Bench Vice_ (Autodesk Fusion 360 archive; units mm, degrees)
design "Screw Bar"
Autodesk Fusion 360 part; units mm, degrees
sketch "Sketch1" plane through (0, 0, 0) normal (0, 0, 1) x (1, 0, 0)
  line L0 (0, 0) -> (84, 0)
  line L1 (84, 0) -> (84, 3)
  line L2 (84, 3) -> (94, 3)
  line L3 (94, 3) -> (94, 5)
  line L4 (94, 5) -> (-10, 5)
  line L5 (-10, 5) -> (-10, 3)
  line L6 (-10, 3) -> (0, 3)
  line L7 (0, 3) -> (0, 0)
  constraint coincident L0.start L7.end
  constraint horizontal L0
  constraint perpendicular L0 L1
  constraint perpendicular L1 L2
  constraint vertical L3
  constraint perpendicular L3 L4
  constraint perpendicular L4 L5
  constraint perpendicular L5 L6
revolve "Revolve1" add sketch "Sketch1" angle 360 about axis through (94, 5, 0) along (-1, 0, 0)

design "Untitled"
Autodesk Fusion 360 part; units mm, degrees
sketch "Sketch1" plane through (0, 0, 0) normal (0, 1, 0) x (1, 0, 0)
  line L0 (0, 0) -> (144, 0)
  line L1 (144, 0) -> (144, -16)
  line L2 (144, -16) -> (0, -16)
  line L3 (0, -16) -> (0, 0)
  line L4 (0, -16) -> (26, -16)
  line L5 (26, -16) -> (26, -52)
  line L6 (26, -52) -> (16, -52)
  line L7 (0, -36) -> (0, -16)
  line L8 (144, -16) -> (122, -16)
  line L9 (122, -16) -> (122, -52)
  line L10 (122, -52) -> (144, -52)
  line L11 (144, -52) -> (144, -16)
  line L12 (0, -36) -> (16, -52)
  dimension "d1" = 144
  dimension "d2" = 16
  dimension "d3" = 26
  dimension "d5" = 22
  dimension "d6" = 36
  constraint horizontal L0
  constraint vertical L1
  constraint horizontal L2
  constraint vertical L3
  constraint coincident L0.start L3.end
  constraint horizontal L4
  constraint vertical L5
  constraint horizontal L6
  constraint vertical L7
  constraint horizontal L8
  constraint vertical L9
  constraint horizontal L10
  constraint vertical L11
  measures "d1" distance of L0.start L0.end
  measures "d2" distance of L0.start L2.end
  measures "d3" distance of L2.end L4.end
  measures "d5" distance of L1.end L8.end
  measures "d6" distance of L1.end L10.end
extrude "Extrude1" add sketch "Sketch1" along normal blind 64 makes body 1
sketch "Sketch2" plane through (144, 0, 0) normal (1, 0, 0) x (0, 1, 0)
  line L0 (0, 52) -> (0, 0)
  line L1 (0, 0) -> (64, 0)
  line L2 (64, 0) -> (64, 52)
  line L3 (64, 52) -> (0, 52)
  line L4 (16, 9) -> (16, 0)
  line L5 (48, 9) -> (48, 0)
  line L6 (16, 0) -> (16, 9)
  line L7 (24, 16) -> (40, 16)
  line L8 (24, 16) -> (24, 9)
  line L9 (40, 16) -> (40, 9)
  line L10 (16, 9) -> (24, 9)
  line L11 (40, 9) -> (48, 9)
  constraint coincident L1 L4.end
  constraint perpendicular L1 L4
  constraint coincident L1 L5.end
  constraint perpendicular L1 L5
  constraint perpendicular L5 L7
  constraint perpendicular L1 L8
  constraint perpendicular L1 L9
  constraint perpendicular L2 L10
  constraint collinear L10 L11
extrude "Extrude2" cut sketch "Sketch2" against normal blind 170 contours L1 L4 L5 L6 L7 L8 L9 L10 L11 bodies 1
sketch "Sketch3" plane through (144, 0, 0) normal (1, 0, 0) x (0, 1, 0)
  line L0 (48, 9) -> (48, 0)
  line L1 (48, 0) -> (64, 0)
  line L2 (64, 0) -> (64, 52)
  line L3 (64, 52) -> (0, 52)
  line L4 (0, 52) -> (0, 0)
  line L5 (0, 0) -> (16, 0)
  line L6 (16, 0) -> (16, 9)
  line L7 (16, 9) -> (24, 9)
  line L8 (24, 9) -> (24, 16)
  line L9 (24, 16) -> (40, 16)
  line L10 (40, 16) -> (40, 9)
  line L11 (40, 9) -> (48, 9)
  circle A0 centre (32, 36) radius 8
  line L12 (46.5857, 42.577) -> (58.5699, 16)
  line L13 (17.4559, 42.6685) -> (4.6049, 16)
  arc A1 (46.5857, 42.577) -> (17.4559, 42.6685) centre (32, 36) ccw
  line L14 (24, 16) -> (40, 16)
  line L15 (4.6049, 16) -> (0, 16)
  line L16 (58.5699, 16) -> (64, 16)
  dimension "d22" = 50
  dimension "d23" = 25.728
  dimension "d25" = 24.272
  constraint coincident L8.end L9.start
  constraint perpendicular L2 L14
  constraint concentric A0 A1
  constraint tangent L12 A1
  constraint coincident L12.end L14
  constraint perpendicular L4 L15
  constraint coincident L2 L16.end
  constraint perpendicular L2 L16
  measures "d22" angle of L12 L13
  measures "d23" angle of L4 L13
  measures "d25" angle of L2 L12
extrude "Extrude3" cut sketch "Sketch3" against normal blind 35 contours L2 L3 L12 A1 L16 | L3 L4 L13 A1 L15 | A0 bodies 1
fillet "Fillet1" radius 3 1 edges at (133, 4.6049, 16) on bodies 1
fillet "Fillet2" radius 3 1 edges at (133, 58.5699, 16) on bodies 1
sketch "Sketch4" plane through (0, 0, 0) normal (0, 1, 0) x (1, 0, 0)
hole "Hole1" at (105.944, 10.2209, 0) direction (0, 0, 1) diameter 6 depth 10 tip angle 118 bodies 1
pattern_linear "R-Pattern1" count 2 spacing 70 along (-1, 0, 0) count 2 spacing 44 along (0, 1, 0) of "Hole1"
sketch "Sketch5" plane through (26, 0, 0) normal (1, 0, 0) x (0, 1, 0)
  line L0 (0, 52) -> (0, 16)
  line L1 (0, 16) -> (24, 16)
  line L2 (40, 16) -> (64, 16)
  line L3 (64, 16) -> (64, 52)
  line L4 (64, 52) -> (0, 52)
  circle A0 centre (32, 34) radius 6
  circle A1 centre (32, 34) radius 16.0001
  line L5 (20.7258, 45.3532) -> (0, 24.7716)
  line L6 (44.2406, 44.3039) -> (64, 24.682)
  line L7 (24, 16) -> (24, 9)
  line L8 (24, 9) -> (40, 9)
  line L9 (40, 9) -> (40, 16)
  dimension "d47" = 45.2
  dimension "d48" = 45.2
  constraint concentric A0 A1
  constraint tangent A1 L5
  constraint coincident A1 L6.start
  constraint coincident A1 L5.start
  constraint coincident L0 L5.end
  constraint coincident L3 L6.end
  constraint coincident L1.end L7.start
  constraint perpendicular L1 L7
  constraint perpendicular L7 L8
  constraint coincident L2.start L9.end
  measures "d47" angle of L0 L5
  measures "d48" angle of L3 L6
sketch "Sketch6" plane through (0, 0, 9) normal (0, 0, -1) x (1, 0, 0)
sketch "Sketch7" plane through (-18, 0, 18) normal (-0.707107, 0, 0.707107) x (0, -1, 0)
  line L0 (0, 25.4558) -> (0, 48.0833)
  line L1 (0, 48.0833) -> (-64, 48.0833)
  line L2 (-64, 48.0833) -> (-64, 25.4558)
  line L3 (-64, 25.4558) -> (0, 25.4558)
sketch "Sketch8" plane through (0, 0, 11) normal (0, 0, -1) x (1, 0, 0)
extrude "Extrude1'" add 1 faces at (26, 34.6667, 40) along direction (1, 0, 0) blind 10 separate body on bodies 1 makes body 2 in component "Component"
sketch "Sketch9" plane through (36, 0, 0) normal (1, 0, 0) x (0, 1, 0)
  line L0 (0, 52) -> (0, 16)
  line L1 (0, 16) -> (64, 16)
  line L2 (64, 16) -> (64, 52)
  line L3 (64, 52) -> (0, 52)
  circle A0 centre (32, 36) radius 6
  circle A1 centre (32, 36) radius 16
  line L4 (0, 16) -> (0, 26)
  line L5 (0, 26) -> (4, 26)
  line L6 (4, 26) -> (19.3557, 45.8041)
  line L7 (60, 26) -> (44.6443, 45.8041)
  line L8 (64, 26) -> (60, 26)
  line L9 (64, 16) -> (64, 26)
  line L10 (24, 16) -> (24, 9)
  line L11 (24, 9) -> (40, 9)
  line L12 (40, 9) -> (40, 16)
  dimension "d81" = 12
  dimension "d82" = 32
  constraint concentric A0 A1
  constraint coincident L0.end L1.start
  constraint perpendicular L1 L4
  constraint horizontal L5
  constraint coincident A1 L6.end
  constraint tangent A1 L6
  constraint coincident L1 L10.start
  constraint perpendicular L1 L10
  constraint perpendicular L10 L11
  constraint coincident L1 L12.end
  constraint perpendicular L1 L12
  measures "d81" diameter of A0
  measures "d82" diameter of A1
extrude "Extrude2'" add sketch "Sketch9" along normal blind 32 contours L0 L1 L2 A1 L4 L5 L6 L7 L8 L9 | A1 | L1 L10 L11 L12 bodies 2 in component "Component"
sketch "Sketch10" plane through (26, 0, 0) normal (1, 0, 0) x (0, 1, 0)
component "Component" placed x (1, 0, 0) y (0, 1, 0) z (0, 0, 1) at (6, 0, 0)
hidden bodies 1

design "Bench Vice" references "Untitled", "Bench Vice", "Jaw Screw", "Screw Bar"
Autodesk Fusion 360 part; units mm, degrees
sketch "Sketch1" plane through (0, 0, 0) normal (0, 1, 0) x (1, 0, 0)
  line L0 (0, 0) -> (144, 0)
  line L1 (144, 0) -> (144, -16)
  line L2 (144, -16) -> (0, -16)
  line L3 (0, -16) -> (0, 0)
  line L4 (0, -16) -> (26, -16)
  line L5 (26, -16) -> (26, -52)
  line L6 (26, -52) -> (16, -52)
  line L7 (0, -36) -> (0, -16)
  line L8 (144, -16) -> (122, -16)
  line L9 (122, -16) -> (122, -52)
  line L10 (122, -52) -> (144, -52)
  line L11 (144, -52) -> (144, -16)
  line L12 (0, -36) -> (16, -52)
  dimension "d1" = 144
  dimension "d2" = 16
  dimension "d3" = 26
  dimension "d5" = 22
  dimension "d6" = 36
  constraint horizontal L0
  constraint vertical L1
  constraint horizontal L2
  constraint vertical L3
  constraint coincident L0.start L3.end
  constraint horizontal L4
  constraint vertical L5
  constraint horizontal L6
  constraint vertical L7
  constraint horizontal L8
  constraint vertical L9
  constraint horizontal L10
  constraint vertical L11
  measures "d1" distance of L0.start L0.end
  measures "d2" distance of L0.start L2.end
  measures "d3" distance of L2.end L4.end
  measures "d5" distance of L1.end L8.end
  measures "d6" distance of L1.end L10.end
extrude "Extrude1" add sketch "Sketch1" along normal blind 64
sketch "Sketch2" plane through (144, 0, 0) normal (1, 0, 0) x (0, 1, 0)
  line L0 (0, 52) -> (0, 0)
  line L1 (0, 0) -> (64, 0)
  line L2 (64, 0) -> (64, 52)
  line L3 (64, 52) -> (0, 52)
  line L4 (16, 9) -> (16, 0)
  line L5 (48, 9) -> (48, 0)
  line L6 (16, 0) -> (16, 9)
  line L7 (24, 16) -> (40, 16)
  line L8 (24, 16) -> (24, 9)
  line L9 (40, 16) -> (40, 9)
  line L10 (16, 9) -> (24, 9)
  line L11 (40, 9) -> (48, 9)
  constraint coincident L1 L4.end
  constraint perpendicular L1 L4
  constraint coincident L1 L5.end
  constraint perpendicular L1 L5
  constraint perpendicular L5 L7
  constraint perpendicular L1 L8
  constraint perpendicular L1 L9
  constraint perpendicular L2 L10
  constraint collinear L10 L11
extrude "Extrude2" cut sketch "Sketch2" against normal blind 170 contours L1 L4 L5 L6 L7 L8 L9 L10 L11
sketch "Sketch3" plane through (144, 0, 0) normal (1, 0, 0) x (0, 1, 0)
  line L0 (48, 9) -> (48, 0)
  line L1 (48, 0) -> (64, 0)
  line L2 (64, 0) -> (64, 52)
  line L3 (64, 52) -> (0, 52)
  line L4 (0, 52) -> (0, 0)
  line L5 (0, 0) -> (16, 0)
  line L6 (16, 0) -> (16, 9)
  line L7 (16, 9) -> (24, 9)
  line L8 (24, 9) -> (24, 16)
  line L9 (24, 16) -> (40, 16)
  line L10 (40, 16) -> (40, 9)
  line L11 (40, 9) -> (48, 9)
  circle A0 centre (32, 36) radius 8
  line L12 (46.5857, 42.577) -> (58.5699, 16)
  line L13 (17.4559, 42.6685) -> (4.6049, 16)
  arc A1 (46.5857, 42.577) -> (17.4559, 42.6685) centre (32, 36) ccw
  line L14 (24, 16) -> (40, 16)
  line L15 (4.6049, 16) -> (0, 16)
  line L16 (58.5699, 16) -> (64, 16)
  dimension "d22" = 50
  dimension "d23" = 25.728
  dimension "d25" = 24.272
  constraint coincident L8.end L9.start
  constraint perpendicular L2 L14
  constraint concentric A0 A1
  constraint tangent L12 A1
  constraint coincident L12.end L14
  constraint perpendicular L4 L15
  constraint coincident L2 L16.end
  constraint perpendicular L2 L16
  measures "d22" angle of L12 L13
  measures "d23" angle of L4 L13
  measures "d25" angle of L2 L12
extrude "Extrude3" cut sketch "Sketch3" against normal blind 35 contours L2 L3 L12 A1 L16 | L3 L4 L13 A1 L15 | A0
fillet "Fillet1" radius 3 1 edges at (133, 4.6049, 16)
fillet "Fillet2" radius 3 1 edges at (133, 58.5699, 16)
sketch "Sketch4" plane through (0, 0, 0) normal (0, 1, 0) x (1, 0, 0)
hole "Hole1" at (105.944, 10.2209, 0) direction (0, 0, 1) diameter 6 depth 10 tip angle 118
pattern_linear "R-Pattern1" count 2 spacing 70 along (-1, 0, 0) count 2 spacing 44 along (0, 1, 0) of "Hole1"
sketch "Sketch5" plane through (26, 0, 0) normal (1, 0, 0) x (0, 1, 0)
  line L0 (0, 52) -> (0, 16)
  line L1 (0, 16) -> (24, 16)
  line L2 (40, 16) -> (64, 16)
  line L3 (64, 16) -> (64, 52)
  line L4 (64, 52) -> (0, 52)
  circle A0 centre (32, 34) radius 6
  circle A1 centre (32, 34) radius 16.0001
  line L5 (20.7258, 45.3532) -> (0, 24.7716)
  line L6 (44.2406, 44.3039) -> (64, 24.682)
  line L7 (24, 16) -> (24, 9)
  line L8 (24, 9) -> (40, 9)
  line L9 (40, 9) -> (40, 16)
  dimension "d47" = 45.2
  dimension "d48" = 45.2
  constraint concentric A0 A1
  constraint tangent A1 L5
  constraint coincident A1 L6.start
  constraint coincident A1 L5.start
  constraint coincident L0 L5.end
  constraint coincident L3 L6.end
  constraint coincident L1.end L7.start
  constraint perpendicular L1 L7
  constraint perpendicular L7 L8
  constraint coincident L2.start L9.end
  measures "d47" angle of L0 L5
  measures "d48" angle of L3 L6
sketch "Sketch6" plane through (0, 0, 9) normal (0, 0, -1) x (1, 0, 0)
sketch "Sketch7" plane through (-18, 0, 18) normal (-0.707107, 0, 0.707107) x (0, -1, 0)
  line L0 (0, 25.4558) -> (0, 48.0833)
  line L1 (0, 48.0833) -> (-64, 48.0833)
  line L2 (-64, 48.0833) -> (-64, 25.4558)
  line L3 (-64, 25.4558) -> (0, 25.4558)
sketch "Sketch8" plane through (0, 0, 11) normal (0, 0, -1) x (1, 0, 0)
sketch "Sketch9" plane through (36, 0, 0) normal (1, 0, 0) x (0, 1, 0)
  line L0 (0, 52) -> (0, 16)
  line L1 (0, 16) -> (64, 16)
  line L2 (64, 16) -> (64, 52)
  line L3 (64, 52) -> (0, 52)
  circle A0 centre (32, 36) radius 6
  circle A1 centre (32, 36) radius 16
  line L4 (0, 16) -> (0, 26)
  line L5 (0, 26) -> (4, 26)
  line L6 (4, 26) -> (19.3557, 45.8041)
  line L7 (60, 26) -> (44.6443, 45.8041)
  line L8 (64, 26) -> (60, 26)
  line L9 (64, 16) -> (64, 26)
  line L10 (24, 16) -> (24, 9)
  line L11 (24, 9) -> (40, 9)
  line L12 (40, 9) -> (40, 16)
  dimension "d81" = 12
  dimension "d82" = 32
  constraint concentric A0 A1
  constraint coincident L0.end L1.start
  constraint perpendicular L1 L4
  constraint horizontal L5
  constraint coincident A1 L6.end
  constraint tangent A1 L6
  constraint coincident L1 L10.start
  constraint perpendicular L1 L10
  constraint perpendicular L10 L11
  constraint coincident L1 L12.end
  constraint perpendicular L1 L12
  measures "d81" diameter of A0
  measures "d82" diameter of A1
sketch "Sketch10" plane through (26, 0, 0) normal (1, 0, 0) x (0, 1, 0)

design "Jaw Screw"
Autodesk Fusion 360 part; units mm, degrees
sketch "Sketch1" plane through (0, 0, 0) normal (0, 0, 1) x (1, 0, 0)
  line L0 (0, 0) -> (82, 0)
  line L1 (82, 0) -> (82, 2)
  line L2 (82, 2) -> (92, 2)
  line L3 (92, 2) -> (92, 0)
  line L4 (92, 0) -> (116, 0)
  line L5 (116, 0) -> (116, 9)
  line L6 (116, 9) -> (-22, 9)
  line L7 (0, 0) -> (0, 2)
  line L8 (0, 2) -> (-9, 2)
  line L9 (-9, 2) -> (-9, 4)
  line L10 (-9, 4) -> (-15, 4)
  line L11 (-15, 4) -> (-15, 2)
  line L12 (-15, 2) -> (-22, 2)
  line L13 (-22, 9) -> (-22, 2)
  line L14 (-35.7467, 9) -> (140.9529, 9) construction
  constraint coincident L0.start L7.start
  constraint horizontal L0
  constraint perpendicular L0 L1
  constraint perpendicular L1 L2
  constraint perpendicular L2 L3
  constraint perpendicular L3 L4
  constraint perpendicular L4 L5
  constraint perpendicular L5 L6
  constraint perpendicular L0 L7
  constraint perpendicular L7 L8
  constraint perpendicular L8 L9
  constraint perpendicular L9 L10
  constraint perpendicular L10 L11
  constraint perpendicular L11 L12
  constraint perpendicular L5 L14
revolve "Revolve1" add sketch "Sketch1" angle 360 about axis through (-35.7467, 9, 0) along (1, 0, 0) in component "Jaw Screw"
move_body "Move1" bodies 1 to x (1, 0, 0) y (0, 1, 0) z (0, 0, 1) at (-27.2122, -28.043, -0.8308) in component "Jaw Screw"
hole "Hole1" at (76.7878, -19.043, 8.1692) direction (0, 0, -1) diameter 6 depth 21 tip angle 118 in component "Jaw Screw"
delete_face "DeleteFace1" 1 faces at (74.5046, -20.9889, -3.7681) in component "Jaw Screw"
hole "Hole2" at (76.7878, -19.043, 8.1692) direction (0, 0, -1) diameter 6 depth 20 tip angle 118 in component "Jaw Screw"
component "Jaw Screw" placed x (1, 0, 0) y (0, 1, 0) z (0, 0, 1) at (0, 0, 0)
